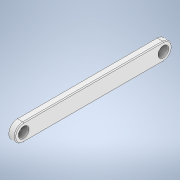
# Autodesk Inventor part: base4
Saved by Autodesk Inventor 2022 (Build 260153000, 153)
## iProperties
Created: 2022-06-14
Part Number: base4
Material: ABS プラスチック
Document SubType Name: Modeling
Designer: yuto6
Density: 1.06 g/cm^3
Appearance: 滑らか - 白
Author: yuto6
Autodesk Inventor part; units mm, degrees
ref_plane "YZ Plane" through (0, 0, 0) normal (1, 0, 0) x (0, 1, 0)
ref_plane "XZ Plane" through (0, 0, 0) normal (0, 1, 0) x (-1, 0, 0)
ref_plane "XY Plane" through (0, 0, 0) normal (0, 0, 1) x (1, 0, 0)
sketch "スケッチ1" plane through (0, 0, 0) normal (1, 0, 0) x (0, 1, 0)
  line L0 (10, -90) -> (-10, -90)
  line L1 (-10, -90) -> (-10, 90)
  line L2 (-10, 90) -> (10, 90)
  line L3 (10, 90) -> (10, -90)
  line L4 (10, -90) -> (-10, 90) construction
  line L5 (-10, -90) -> (10, 90) construction
  point P0 (0, 0)
  dimension "d0" = 180
  dimension "d1" = 20
  constraints: 12 end point, 2 midpoint, 2 parallel, 1 horizontal, 1 perpendicular
  measures "d0" distance of L2.end L0.start
  measures "d1" distance of L1.end L2.end
extrude "押し出し1" add sketch "スケッチ1" along normal blind 8
sketch "スケッチ2" plane through (8, 0, 0) normal (1, 0, 0) x (0, 0, -1)
  line L0 (-90, 10) -> (-90, -10) projected
  line L1 (90, -10) -> (90, 10) projected
  point P0 (0, 0)
  point P1 (-80, 0)
  point P2 (80, 0)
  dimension "d4" = 10
  dimension "d14" = 10
  measures "d4" distance from line of L0 point (-80, 0)
  measures "d14" distance from line of L1 point (80, 0)
hole "穴1" at (8, 0, 80) at (8, 0, -80) direction (-1, 0, 0) diameter 12.3 end through all
fillet "フィレット1" radius 10 4 edges at (4, 10, 90) (4, -10, 90) (4, 10, -90) (4, -10, -90)
fillet "フィレット2" radius 1 8 edges at (0, 7.0712, -87.0712) (0, 10, 0) (0, 7.0712, 87.0712) (0, -10, 0) (8, 7.0712, -87.0712) (8, 10, 0) (8, 7.0712, 87.0712) (8, -10, 0)
equation "\"d14\" = d4"
